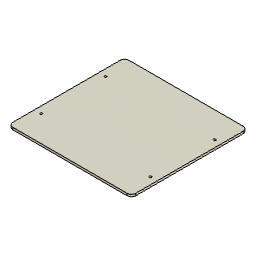
white_plate v3 (Autodesk Fusion 360 design; units mm, degrees)
Autodesk Fusion 360 part; units mm, degrees
sketch "Sketch1" plane through (0, 0, 0) normal (0, 0, 1) x (1, 0, 0)
  line L0 (0, 0) -> (180, 0)
  line L1 (180, 0) -> (180, 170)
  line L2 (180, 170) -> (0, 170)
  line L3 (0, 170) -> (0, 0)
  dimension "d1" = 180
  dimension "d2" = 170
  constraint horizontal L0
  constraint vertical L1
  constraint horizontal L2
  constraint vertical L3
  constraint coincident L0.start L3.end
  measures "d1" distance of L0.start L0.end
  measures "d2" distance of L0.start L2.end
extrude "Extrude1" add sketch "Sketch1" along normal blind 3.175
fillet "Fillet1" radius 6.35 2 edges at (0, 0, 1.5875) (180, 0, 1.5875)
fillet "Fillet2" radius 6.35 2 edges at (0, 170, 1.5875) (180, 170, 1.5875)
sketch "Sketch2" plane through (0, 0, 3.175) normal (0, 0, 1) x (-1, 0, 0)
  arc A0 (-180, -163.65) -> (-173.65, -170) centre (-173.65, -163.65) ccw
  line L0 (-173.65, -170) -> (-6.35, -170)
  arc A1 (-6.35, -170) -> (0, -163.65) centre (-6.35, -163.65) ccw
  line L1 (0, -163.65) -> (0, -6.35)
  arc A2 (0, -6.35) -> (-6.35, 0) centre (-6.35, -6.35) ccw
  line L2 (-6.35, 0) -> (-173.65, 0)
  arc A3 (-173.65, 0) -> (-180, -6.35) centre (-173.65, -6.35) ccw
  line L3 (-180, -6.35) -> (-180, -163.65)
  circle A4 centre (-10, -38) radius 1.5875
  circle A5 centre (-170, -38) radius 1.5875
  circle A6 centre (-10, -132) radius 1.5875
  circle A7 centre (-170, -132) radius 1.5875
  dimension "d9" = 3.175
  dimension "d10" = 3.175
  dimension "d11" = 3.175
  dimension "d12" = 3.175
  dimension "d13" = 94
  dimension "d14" = 94
  dimension "d15" = 10
  dimension "d16" = 10
  dimension "d17" = 38
  dimension "d18" = 38
  dimension "d19" = 10
  dimension "d20" = 10
  measures "d9" diameter of A6
  measures "d10" diameter of A7
  measures "d11" diameter of A4
  measures "d12" diameter of A5
  measures "d13" vertical distance of A4.centre A6.centre
  measures "d14" vertical distance of A5.centre A7.centre
  measures "d15" distance of L1 A6.centre
  measures "d16" distance of L1 A4.centre
  measures "d17" distance of L0 A6.centre
  measures "d18" distance of L0 A7.centre
  measures "d19" distance of L3 A7.centre
  measures "d20" distance of L3 A5.centre
extrude "Extrude2" cut sketch "Sketch2" against normal blind 10 contours A4 | A5 | A6 | A7
